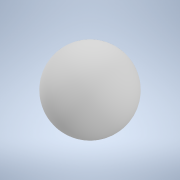
# Autodesk Inventor part: Ball
Saved by Autodesk Inventor 2020.4 (Build 244396000, 396)
## iProperties
Created: 2022-01-05
Part Number: Ball
Material: 一般
Document SubType Name: Modeling
Designer: Masato Kubotera
Appearance: 既定
Surface Area: 530.929 cm^2
Volume: 1150.35 cm^3
Author: Masato Kubotera
Autodesk Inventor part; units mm, degrees
ref_plane "YZ Plane" through (0, 0, 0) normal (1, 0, 0) x (0, 1, 0)
ref_plane "XZ Plane" through (0, 0, 0) normal (0, 1, 0) x (-1, 0, 0)
ref_plane "XY Plane" through (0, 0, 0) normal (0, 0, 1) x (1, 0, 0)
sketch "スケッチ1" plane through (0, 0, 0) normal (0, 0, 1) x (1, 0, 0)
  line L0 (-65, 0) -> (65, 0)
  arc A0 (65, 0) -> (-65, 0) centre (0, 0) ccw
  dimension "d0" = 130
  constraints: 2 coincident, 2 end point, 2 point on circle, 1 centre point, 1 horizontal, 1 midpoint
  measures "d0" distance of L0.start L0.end
revolve "回転1" add sketch "スケッチ1" angle 360 about axis through (-65, 0, 0) along (1, 0, 0)
